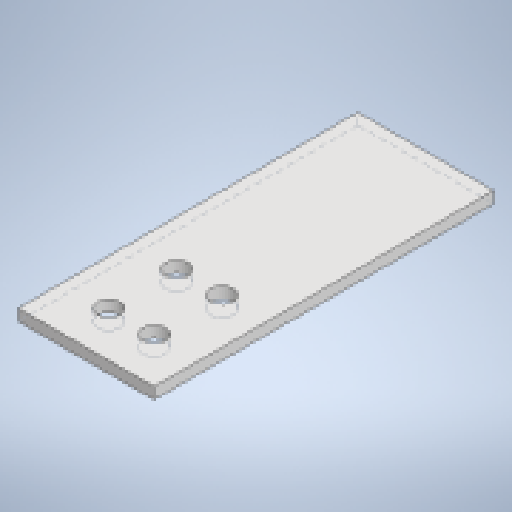
# Autodesk Inventor part: body-1
Saved by Autodesk Inventor 2025 (Build 290162000, 162)
## iProperties
Created: 2026-01-27
Part Number: body-1
Material: 一般
Document SubType Name: Modeling
Designer: mahhy
Density: 1 g/cm^3
Appearance: 既定
Author: mahhy
Autodesk Inventor part; units mm, degrees
ref_plane "YZ Plane" through (0, 0, 0) normal (1, 0, 0) x (0, 1, 0)
ref_plane "XZ Plane" through (0, 0, 0) normal (0, 1, 0) x (-1, 0, 0)
ref_plane "XY Plane" through (0, 0, 0) normal (0, 0, 1) x (1, 0, 0)
sketch "底面スケッチ" plane through (0, 0, 0) normal (0, 1, 0) x (-1, 0, 0)
  line L0 (0, 0) -> (60, 0)
  line L1 (60, 0) -> (60, -150)
  line L2 (60, -150) -> (0, -150)
  line L3 (0, -150) -> (0, 0)
  dimension "d0" = 60
  dimension "d1" = 150
  constraints: 8 end point, 2 parallel, 1 horizontal, 1 perpendicular
  measures "d0" distance of L1.end L2.end
  measures "d1" distance of L0.end L1.end
extrude "底面" add sketch "底面スケッチ" along normal blind 6
sketch "スケッチ2" plane through (0, 6, 0) normal (0, 1, 0) x (1, 0, 0)
  line L0 (-50, 10) -> (-20, 10)
  line L1 (-20, 10) -> (-20, 60)
  line L2 (-20, 60) -> (-50, 60)
  line L3 (-50, 60) -> (-50, 10)
  line L4 (-60, 0) -> (0, 0) projected
  line L5 (-60, 150) -> (-60, 0) projected
  dimension "d12" = 30
  dimension "d13" = 50
  dimension "d14" = 10
  dimension "d15" = 10
  constraints: 8 end point, 2 parallel, 1 horizontal, 1 perpendicular
  measures "d12" distance of L2.end L1.end
  measures "d13" distance of L1.end L0.end
  measures "d14" distance between parallel lines of L4 L0
  measures "d15" distance between parallel lines of L5 L3
extrude "溝" cut sketch "スケッチ2" against normal blind 2
